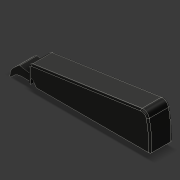
# Autodesk Inventor part: black_key
Saved by Autodesk Inventor 2020.2 (Build 242310000, 310)
## iProperties
Created: 2020-07-05
Part Number: black_key
Material: PLA (Black, 3D Printed)
Document SubType Name: Modeling
Designer: isaac
Density: 1 g/cm^3
Appearance: PLA (Black)
Mass: 7.16889 g
Surface Area: 30.1151 cm^2
Volume: 7.16889 cm^3
Author: isaac
Autodesk Inventor part; units mm, degrees
ref_plane "YZ Plane" through (0, 0, 0) normal (1, 0, 0) x (0, 1, 0)
ref_plane "XZ Plane" through (0, 0, 0) normal (0, 1, 0) x (-1, 0, 0)
ref_plane "XY Plane" through (0, 0, 0) normal (0, 0, 1) x (1, 0, 0)
sketch "Profile Sketch" plane through (0, 0, 0) normal (1, 0, 0) x (0, 1, 0)
  line L0 (-2, 2.1422) -> (-2, 54.9636)
  arc A0 (11.247, 53.8378) -> (-2, 54.9636) centre (0, 0) ccw
  line L1 (13.6019, 50.4669) -> (6.1877, -0.2171)
  line L2 (-2, 2.1422) -> (0.3454, 0.4906)
  arc A1 (0, -0.6) -> (0.3454, 0.4906) centre (0, 0) ccw
  line L3 (0, -0.6) -> (-2, -0.6)
  line L4 (-2, -0.6) -> (-2, -8.1183)
  line L5 (-2, -8.1183) -> (-4.7049, -10.8232)
  line L6 (-4.7781, -11.25) -> (-2, -11.25)
  line L7 (4.7035, -1.5) -> (1.4679, -1.5)
  line L8 (1, -1.5) -> (2, -7)
  line L9 (2, -7) -> (-2, -11.25)
  line L10 (-2, 4.4659) -> (1.4394, 2.0441)
  arc A2 (2.3633, -0.8155) -> (1.4394, 2.0441) centre (0, 0) ccw
  line L11 (2.3633, -0.8155) -> (-0.027, -0.6)
  arc A3 (4.7035, -1.5) -> (6.1877, -0.2171) centre (4.7035, 0) ccw
  arc A4 (13.6019, 50.4669) -> (11.247, 53.8378) centre (10.6335, 50.9012) ccw
  line L12 (4.7035, 0) -> (0, 0) construction
  line L13 (1.4679, -1.5) -> (-2, -1.5)
  arc A5 (-4.7049, -10.8232) -> (-4.5281, -11.25) centre (-4.5281, -11) ccw
  line L14 (-4.7781, -11.25) -> (-4.7781, -11) construction
  point P0 (14, 53.1883)
  point P1 (6, -1.5)
  dimension "d0" = 0.6
  dimension "d2" = 45
  dimension "d4" = 55
  dimension "d7" = 54.848
  dimension "d8" = 2.5
  dimension "d9" = 5.152
  dimension "d10" = 2
  dimension "d11" = 16
  dimension "d12" = 8
  dimension "d13" = 1.5
  dimension "d14" = 3
  dimension "d20" = 2.7781
  dimension "d26" = 11
  dimension "d27" = 0.25
  dimension "d28" = 7
  dimension "d30" = 1
  dimension "d31" = 3
  constraints: 30 end point, 14 point on circle, 11 tangent, 10 point on line, 6 centre point, 5 horizontal, 3 coincident, 3 vertical, 1 parallel
  measures "d0" radius of A1
  measures "d2" angle of L4 L5
  measures "d4" radius of A0
  measures "d7" angle of L2 L0
  measures "d8" radius of A2
  measures "d9" angle of L3 L11
  measures "d10" distance from line of point (0, 0) L0
  measures "d11" distance from line of L0 point (14, 53.188)
  measures "d12" distance from line of L4 point (6, -1.5)
  measures "d13" radius of A3
  measures "d14" radius of A4
  measures "d20" distance from line of L4 L6.start
  measures "d26" vertical distance of point (0, 0) A5.centre
  measures "d27" radius of A5
  measures "d28" vertical distance of point (0, 0) L8.end
  measures "d30" horizontal distance of L8.start L8.end
  measures "d31" distance of L13.end L8.start
extrude "Main Key" add sketch "Profile Sketch" along normal mid plane 10.275 contours L0 L10 A2 L11 L3 A1 L2 | L0 A0 A4 L1 A3 L7 L13 L4 L3 L11 A2 L10
extrude "Extrusion2" add sketch "Profile Sketch" along normal mid plane 8 contours L13 L8 L9 L6 A5 L5 L4
fillet "Fillet1" radius 0.7 10 edges at (-5.1375, 5.6844, -1.1348) (-5.1375, 1.3517, -1.5) (-5.1375, 13.0928, 52.6193) (-5.1375, 4.6576, 54.8024) (-5.1375, 9.8948, 25.1249) (5.1375, 13.0928, 52.6193) (5.1375, 4.6576, 54.8024) (5.1375, 5.6844, -1.1348) (5.1375, 1.3517, -1.5) (5.1375, 9.8948, 25.1249)
extrude "Extrusion3" cut sketch "Profile Sketch" along normal mid plane 4.31 contours L0 L10 A2 L11 L3 A1 L2
fillet "Fillet2" radius 5 2 edges at (0, -2, -8.1183) (0, -2, -11.25)
fillet "Fillet3" radius 0.7 1 edges at (0, 2, -7)
equation "\"d0\" = hingeSocketRad"
equation "\"d4\" = blackKeyLength"
equation "\"hingeSocketRad\" = 0.6"
equation "\"blackKeyLength\" = 55"
body "Solid1"
